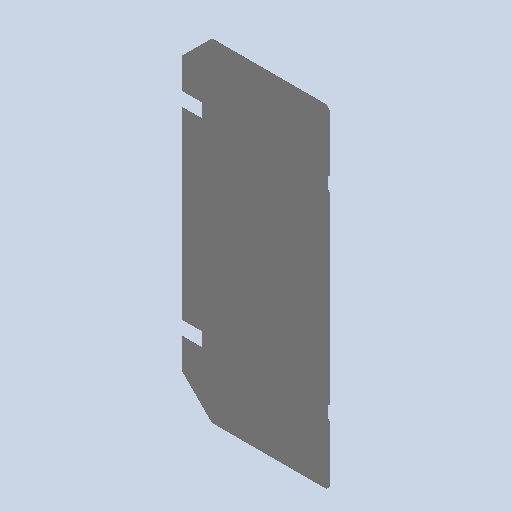
# Autodesk Inventor part: BaseSuperior
Saved by Autodesk Inventor 2022.1 (Build 261234000, 234)
## iProperties
Created: 2021-10-01
Part Number: BaseSuperior
Material: Steel, Alloy
Document SubType Name: Sheet Metal
Designer: Andres
Density: 7.73 g/cm^3
Sheet Metal Rule: Por defecto_mm
Appearance: Semi-Polished
Author: Andres
Autodesk Inventor part; units mm, degrees
ref_plane "YZ Plane" through (0, 0, 0) normal (1, 0, 0) x (0, 1, 0)
ref_plane "XZ Plane" through (0, 0, 0) normal (0, 1, 0) x (-1, 0, 0)
ref_plane "XY Plane" through (0, 0, 0) normal (0, 0, 1) x (1, 0, 0)
sketch "Sketch1" plane through (0, 0, 0) normal (0, 0, 1) x (1, 0, 0)
  line L0 (0, 20) -> (32, 20) construction
  line L1 (32, 20) -> (32, 206.6274) construction
  line L2 (32, 206.6274) -> (2.6274, 236) construction
  line L3 (2.6274, 236) -> (-370.6274, 236) construction
  line L4 (-370.6274, 236) -> (-480, 126.6274) construction
  line L5 (-480, 126.6274) -> (-480, -726.6274) construction
  line L6 (-480, -726.6274) -> (-370.6274, -836) construction
  line L7 (-370.6274, -836) -> (2.6274, -836) construction
  line L8 (2.6274, -836) -> (32, -806.6274) construction
  line L9 (32, -806.6274) -> (32, -620) construction
  line L10 (32, -620) -> (0, -620) construction
  line L11 (0, -793.3726) -> (0, -620) construction
  line L12 (-10.6274, -804) -> (0, -793.3726) construction
  line L13 (-357.3726, -804) -> (-10.6274, -804) construction
  line L14 (-448, -713.3726) -> (-357.3726, -804) construction
  line L15 (-448, 113.3726) -> (-448, -713.3726) construction
  line L16 (-357.3726, 204) -> (-448, 113.3726) construction
  line L17 (-10.6274, 204) -> (-357.3726, 204) construction
  line L18 (0, 193.3726) -> (-10.6274, 204) construction
  line L19 (0, 20) -> (0, 193.3726) construction
  line L20 (-4, -16) -> (-4, 16) construction
  line L21 (-4, 16) -> (-444, 16) construction
  line L22 (-444, 16) -> (-444, -16) construction
  line L23 (-4, -16) -> (-444, -16) construction
  line L24 (-390.9357, 16) -> (-390.9357, -16) construction
  line L25 (-390.9357, -584) -> (-390.9357, -616) construction
  line L26 (-4, -616) -> (-4, -584) construction
  line L27 (-464, -584) -> (-4, -584) construction
  line L28 (-464, -616) -> (-464, -584) construction
  line L29 (-464, -616) -> (-4, -616) construction
  line L30 (32, -20) -> (0, -20) construction
  line L31 (0, -580) -> (0, -20) construction
  line L32 (0, -580) -> (32, -580) construction
  line L33 (32, -580) -> (32, -20) construction
  line L34 (-357.3726, 204) -> (-10.6274, 204)
  line L35 (33, 21) -> (-5, 21)
  line L36 (-5, 21) -> (-5, -21)
  line L37 (-5, -21) -> (33, -21)
  line L38 (33, -21) -> (33, 21)
  line L39 (33, -579) -> (-5, -579)
  line L40 (-5, -579) -> (-5, -621)
  line L41 (-5, -621) -> (33, -621)
  line L42 (33, -621) -> (33, -579)
  line L43 (-385.8175, 21) -> (-481, 21)
  line L44 (-481, 21) -> (-481, -21)
  line L45 (-481, -21) -> (-385.8175, -21)
  line L46 (-385.8175, -21) -> (-385.8175, 21)
  line L47 (-385.8175, -579) -> (-481, -579)
  line L48 (-481, -579) -> (-481, -621)
  line L49 (-481, -621) -> (-385.8175, -621)
  line L50 (-385.8175, -621) -> (-385.8175, -579)
  line L51 (-10.6274, 204) -> (0, 193.3726)
  line L52 (0, 21) -> (0, 193.3726)
  line L53 (0, -21) -> (0, -579)
  line L54 (0, -621) -> (0, -793.3726)
  line L55 (-10.6274, -804) -> (0, -793.3726)
  line L56 (-357.3726, -804) -> (-448, -713.3726)
  line L57 (-448, -621) -> (-448, -713.3726)
  line L58 (-10.6274, -804) -> (-357.3726, -804)
  line L59 (-448, -579) -> (-448, -21)
  line L60 (-448, 21) -> (-448, 113.3726)
  line L61 (-448, 113.3726) -> (-357.3726, 204)
  line L62 (-471.7703, 20) -> (-464.546, 20) construction
  line L63 (-460.946, -20) -> (-288.146, -20) construction
  line L64 (-386.8175, -16) -> (-386.8175, 16) construction
  line L65 (-471.7703, -580) -> (-464.546, -580) construction
  line L66 (-471.7703, -620) -> (-464.546, -620) construction
  line L67 (-386.8175, -616) -> (-386.8175, -584) construction
  point P0 (0, 0)
  dimension "offset" = 1
  dimension "d1" = 1
  dimension "d2" = 1
  dimension "d3" = 1
  dimension "d4" = 1
  dimension "d5" = 1
  dimension "d6" = 1
  dimension "d7" = 1
  dimension "d10" = 1
  dimension "d15" = 1
  dimension "d18" = 1
  dimension "d19" = 1
  dimension "d20" = 1
  dimension "d21" = 1
  dimension "d22" = 1
  dimension "d24" = 1
  measures "offset" distance between parallel lines of L0 L35
  measures "d1" distance between parallel lines of L30 L37
  measures "d2" distance between parallel lines of L20 L36
  measures "d3" distance between parallel lines of L1 L38
  measures "d4" distance between parallel lines of L32 L39
  measures "d5" distance between parallel lines of L33 L42
  measures "d6" distance between parallel lines of L10 L41
  measures "d7" distance between parallel lines of L26 L40
  measures "d10" distance between parallel lines of L5 L44
  measures "d15" distance between parallel lines of L5 L48
  measures "d18" distance between parallel lines of L43 L62
  measures "d19" distance between parallel lines of L46 L64
  measures "d20" distance between parallel lines of L45 L63
  measures "d21" distance between parallel lines of L49 L66
  measures "d22" distance between parallel lines of L67 L50
  measures "d24" distance between parallel lines of L47 L65
extrude "Plate1" add sketch "Sketch1" along normal blind 0.5 contours L34 L51 L52 L35 L36 L37 L53 L39 L40 L41 L54 L55 L58 L56 L57 L49 L50 L47 L59 L45 L46 L43 L60 L61
fillet "Corner Round1" radius 4 8 edges at (-385.8175, 21, 0.25) (-385.8175, -21, 0.25) (-385.8175, -579, 0.25) (-385.8175, -621, 0.25) (-5, -579, 0.25) (-5, -621, 0.25) (-5, -21, 0.25) (-5, 21, 0.25)
equation "\"d1\" = offset"
equation "\"d2\" = offset"
equation "\"d3\" = offset"
equation "\"d4\" = offset"
equation "\"d5\" = offset"
equation "\"d6\" = offset"
equation "\"d7\" = offset"
equation "\"d10\" = offset"
equation "\"d15\" = offset"
equation "\"d18\" = offset"
equation "\"d19\" = offset"
equation "\"d20\" = offset"
equation "\"d21\" = offset"
equation "\"d22\" = offset"
equation "\"d24\" = offset"
equation "\"d16\" = Thickness"
equation "\"BendRadius\" = Thickness"
equation "\"BendReliefWidth\" = Thickness"
equation "\"BendReliefDepth\" = 0.5 * Thickness"
equation "\"CornerReliefSize\" = 4 * Thickness"
equation "\"MinimumRemnant\" = 2 * Thickness"
equation "\"TransitionRadius\" = BendRadius"
equation "\"JacobiRadiusSize\" = BendRadius"
equation "\"GapSize\" = Thickness"
equation "\"Thickness\" = 0.5"
body "Solid1"
